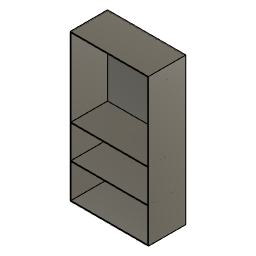
Simpelt skap (Autodesk Fusion 360 design; units mm, degrees)
Autodesk Fusion 360 part; units mm, degrees
note: some values were not read from the file. Set by a fixed rule: which face or edge a step refers to.
sketch "Sketch1" plane through (0, 0, 0) normal (0, 0, 1) x (1, 0, 0)
  line L0 (0, 0) -> (-420, 0)
  line L1 (-420, 0) -> (-420, 200.5342)
  line L2 (-420, 200.5342) -> (0, 200.5342)
  line L3 (0, 200.5342) -> (0, 0)
  line L4 (-413.9466, 194.2871) -> (-6.2935, 194.2871)
  line L5 (-6.2935, 194.2871) -> (-6.2935, 6.8657)
  line L6 (-6.2935, 6.8657) -> (-413.9466, 6.8657)
  line L7 (-413.9466, 6.8657) -> (-413.9466, 194.2871)
  dimension "d1" = 420
  constraint horizontal L0
  constraint vertical L1
  constraint horizontal L2
  constraint vertical L3
  constraint coincident L0.start L3.end
  constraint horizontal L4
  constraint vertical L5
  constraint horizontal L6
  constraint vertical L7
  measures "d1" distance of L0.start L0.end
extrude "Extrude1" add sketch "Sketch1" along normal blind 7 contours L0 L1 L2 L3 | L4 L5 L6 L7
extrude "Extrude2" add 1 faces at (-140, 66.8447, 7) along direction (0, 0, 1) blind 361.615
shell "Shell1" thickness 4 removed faces 1 at (-140, 0, 122.8717)
form "Form1" [no effect]
sketch "Sketch2" plane through (0, 0, 0) normal (0, 0, 1) x (1, 0, 0)
extrude "Extrude3" add 1 faces at (-278.6667, 131.0228, 4) along direction (0, 0, 1) blind 185.509
shell "Shell2" thickness 4 removed faces 1 at (-278.6667, 0, 63.1697)
extrude "Extrude4" add 1 faces at (-140, 66.8447, 368.615) along direction (0, 0, 1) blind 420
shell "Shell3" thickness 4 removed faces 1 at (-278.6667, 0, 647.2817)
sketch "Sketch3" plane through (-416, 0, 0) normal (1, 0, 0) x (0, 1, 0)
  line L0 (0, 368.615) -> (196.5342, 368.615)
  line L1 (196.5342, 368.615) -> (196.5342, 784.615)
  line L2 (196.5342, 784.615) -> (0, 784.615)
  line L3 (0, 784.615) -> (0, 368.615)
  circle A0 centre (98.2671, 724.6245) radius 8.816
extrude "Extrude5" add sketch "Sketch3" along normal blind 411.992 contours A0
